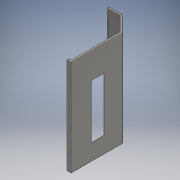
# Autodesk Inventor part: Cover Back
Saved by Autodesk Inventor 2018 (Build 220112000, 112)
## iProperties
Created: 2018-08-07
Part Number: Cover Back
Material: Stainless Steel
Document SubType Name: Modeling
Designer: P301319
Density: 8 g/cm^3
Appearance: Stainless - Brushed
Author: P301319
Autodesk Inventor part; units mm, degrees
ref_plane "YZ Plane" through (0, 0, 0) normal (1, 0, 0) x (0, 1, 0)
ref_plane "XZ Plane" through (0, 0, 0) normal (0, 1, 0) x (-1, 0, 0)
ref_plane "XY Plane" through (0, 0, 0) normal (0, 0, 1) x (1, 0, 0)
sketch "Sketch1" plane through (0, 0, 0) normal (0, 0, 1) x (1, 0, 0)
  line L0 (-347.6, 800) -> (-180, 800)
  line L1 (-180, 800) -> (0, 620)
  line L2 (-180, 800) -> (122.4624, 800) construction
  line L3 (0, 0) -> (0, 620)
  line L4 (0, 0) -> (-50, 0)
  line L5 (-50, -1.6) -> (1.6, -1.6)
  line L6 (1.6, -1.6) -> (1.6, 620.6627)
  line L7 (1.6, 620.6627) -> (-179.3373, 801.6)
  line L8 (-179.3373, 801.6) -> (-347.6, 801.6)
  line L9 (-347.6, 801.6) -> (-347.6, 800)
  line L10 (-50, 0) -> (-50, -1.6)
  dimension "d0" = 167.6
  dimension "d1" = 45
  dimension "d2" = 800
  dimension "d4" = 50
  dimension "d15" = 180
  dimension "d19" = 1.6
  constraints: 22 end point, 3 horizontal, 2 vertical, 1 perpendicular, 3 other
  measures "d0" distance of L0.start L0.end
  measures "d1" angle of L1 L2
  measures "d2" distance from line of L3.start L0
  measures "d4" distance of L3.start L4.end
  measures "d15" distance from line of L3 L0.end
  measures "d19" distance between parallel lines of L1 L7
extrude "Extrusion1" add sketch "Sketch1" along normal blind 1160
sketch "Sketch2" plane through (0, 0, 0) normal (-1, 0, 0) x (0, 0, -1)
  line L0 (-195, -320) -> (-845, -320) construction
  line L1 (-845, -245) -> (-195, -245)
  line L2 (-195, -245) -> (-195, -395)
  line L3 (-195, -395) -> (-845, -395)
  line L4 (-845, -395) -> (-845, -245)
  point P0 (0, 0)
  dimension "d8" = 195
  dimension "d10" = 650
  dimension "d11" = 650
  dimension "d12" = 150
  dimension "d20" = 320
  constraints: 10 end point, 2 horizontal, 2 parallel, 1 midpoint, 1 perpendicular
  measures "d8" horizontal distance of point (0, 0) L0.start
  measures "d10" distance of L0.end L0.start
  measures "d11" distance of L2.end L3.end
  measures "d12" distance of L1.end L2.end
  measures "d20" vertical distance of point (0, 0) L0.start
extrude "Extrusion3" cut sketch "Sketch2" against normal through all
sketch "Sketch3" plane through (0, 0, 0) normal (0, 0, -1) x (-1, 0, 0)
  line L0 (50, 0) -> (0, 0) projected
  line L1 (0, 0) -> (0, 620) projected
  line L2 (0, 620) -> (180, 800) projected
  line L3 (180, 800) -> (347.6, 800) projected
  line L4 (347.6, 780) -> (188.2843, 780)
  line L5 (188.2843, 780) -> (20, 611.7157)
  line L6 (20, 611.7157) -> (20, 20)
  line L7 (20, 20) -> (50, 20)
  line L8 (347.6, 780) -> (347.6, 800)
  line L9 (50, 20) -> (50, 0)
  dimension "d23" = 20
  constraints: 12 end point, 2 vertical, 3 other
  measures "d23" distance between parallel lines of L2 L5
extrude "Extrusion4" add sketch "Sketch3" against normal blind 1.6
sketch "Sketch4" plane through (0, 0, 1160) normal (0, 0, 1) x (1, 0, 0)
  line L0 (0, 0) -> (-50, 0) projected
  line L1 (0, 620) -> (0, 0) projected
  line L2 (-180, 800) -> (0, 620) projected
  line L3 (-347.6, 800) -> (-180, 800) projected
  line L4 (-347.6, 800) -> (-347.6, 780) projected
  line L5 (-347.6, 780) -> (-188.2843, 780) projected
  line L6 (-188.2843, 780) -> (-20, 611.7157) projected
  line L7 (-20, 611.7157) -> (-20, 20) projected
  line L8 (-20, 20) -> (-50, 20) projected
  line L9 (-50, 20) -> (-50, 0) projected
extrude "Extrusion5" add sketch "Sketch4" against normal blind 1.6
sketch "Sketch5" plane through (-347.6, 801.6, 0) normal (-1, 0, 0) x (0, 0, 1)
  line L0 (1.6, -1.6) -> (1.6, -21.6) projected
  line L1 (1.6, -1.6) -> (1158.4, -1.6) projected
  line L2 (1158.4, -21.6) -> (1158.4, -1.6) projected
  line L3 (1.6, -21.6) -> (1158.4, -21.6)
  line L4 (0, 0) -> (0, -180.9373) projected
  point P0 (0, -801.6)
  constraints: 2 end point, 1 perpendicular
extrude "Extrusion6" add sketch "Sketch5" against normal blind 1.6
sketch "Sketch6" plane through (-347.6, 801.6, 0) normal (-1, 0, 0) x (0, 0, 1)
  line L0 (1158.4, -21.6) -> (1.6, -21.6) projected
  line L1 (580, -21.6) -> (580, 0) construction
  line L2 (0, 0) -> (1160, 0) projected
  line L3 (1.6, -1.6) -> (1158.4, -1.6) projected
  line L4 (1.6, -21.6) -> (1.6, -1.6)
  line L5 (3.2, -21.6) -> (3.2, -1.6)
  line L6 (1158.4, -1.6) -> (1158.4, -21.6)
  line L7 (1158.4, -181.6) -> (1158.4, -1.6) projected
  line L8 (1156.8, -1.6) -> (1156.8, -21.6)
  point P0 (0, -801.6)
  dimension "d30" = 1.6
  dimension "d31" = 1.6
  constraints: 10 end point, 4 point on line, 3 perpendicular, 2 midpoint, 1 collinear
  measures "d30" distance between parallel lines of L4 L5
  measures "d31" distance between parallel lines of L6 L8
extrude "Extrusion7" cut sketch "Sketch6" against normal blind 1.6 contours L0 L8 L3 L6 | L0 L4 L3 L5
body "Solid1"
